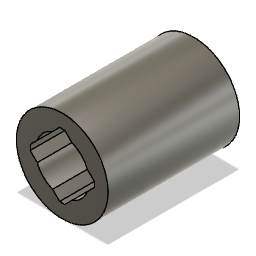
Engine_Pull-Start_Shaft_to_Drill_Adapter (Autodesk Fusion 360 design; units mm, degrees)
Autodesk Fusion 360 part; units mm, degrees
sketch "Sketch3" plane through (0, 0, 0) normal (0, 0, 1) x (1, 0, 0)
  circle A0 centre (0, 0) radius 10.25
  circle A1 centre (0, 0) radius 6
  line L0 (-1, 12.25) -> (1, 12.25)
  line L1 (1, 12.25) -> (3.6855, 9.5645)
  line L2 (-1, 12.25) -> (-3.6855, 9.5645)
  line L3 (-12.25, 1) -> (-9.5645, 3.6855)
  line L4 (-12.25, -1) -> (-9.5645, -3.6855)
  line L5 (-12.25, -1) -> (-12.25, 1)
  line L6 (-1, -12.25) -> (-3.6855, -9.5645)
  line L7 (1, -12.25) -> (3.6855, -9.5645)
  line L8 (1, -12.25) -> (-1, -12.25)
  line L9 (12.25, -1) -> (9.5645, -3.6855)
  line L10 (12.25, 1) -> (9.5645, 3.6855)
  line L11 (12.25, 1) -> (12.25, -1)
  circle A2 centre (0, 0) radius 17.5
  dimension "d1" = 20.5
  dimension "d2" = 12
  dimension "d6" = 2
  dimension "d10" = 360
  dimension "d11" = 35
  constraint coincident A0.centre A1.centre
  constraint coincident A0 L1.end
  constraint concentric A1 A2
  measures "d1" diameter of A0
  measures "d2" diameter of A1
  measures "d6" distance of L0.start L0.end
  measures "d11" diameter of A2
extrude "Extrude1" add sketch "Sketch3" along normal blind 20 contours A1 makes body 1
extrude "Extrude2" add sketch "Sketch3" along normal blind 20 separate body contours A2 makes body 2
cylinder "CylinderPrimitive1" add diameter 35 height -15 placed x (1, 0, 0) y (0, 1, 0) z (0, 0, 1) at (0, 0, 0) bodies 1 2
cylinder "CylinderPrimitive2" add diameter 6 height 30 placed x (0, 1, 0) y (1, 0, 0) z (0, 0, -1) at (0, 0, -15) bodies 1
extrude "Extrude3" cut 1 faces at (-0.9566, -0.2914, 20) along direction (0, 0, -1) up to surface (20 mm away) on bodies 1 bodies 1
scale "Scale1" factor 1.05 about (0, 17.5, -15) bodies 1
extrude "Extrude4" cut 1 faces at (-0.3791, 0.4335, -46.5) along direction (0, 0, 1) up to surface (31.5 mm away) on bodies 1 bodies 1
move_body "Move1" bodies 1 to x (1, 0, 0) y (0, 1, 0) z (0, 0, 1) at (0, 13, 0)
sketch "Sketch7" plane through (0, 0, -15) normal (0, 0, -1) x (-1, 0, 0)
  circle A0 centre (0, 12.125) radius 18.375
  line L0 (-2.7424, 16.875) -> (-5.4848, 12.125)
  line L1 (-5.4848, 12.125) -> (-2.7424, 7.375)
  line L2 (-2.7424, 7.375) -> (2.7424, 7.375)
  line L3 (2.7424, 7.375) -> (5.4848, 12.125)
  line L4 (5.4848, 12.125) -> (2.7424, 16.875)
  line L5 (2.7424, 16.875) -> (-2.7424, 16.875)
  circle A1 centre (0, 12.125) radius 18.375
  point P0 (0, 12.125)
  dimension "d26" = 4.75
  constraint coincident P0 A0.centre
  measures "d26" distance of P0 L5
extrude "Extrude5" add sketch "Sketch7" along normal blind 16 bodies 1
